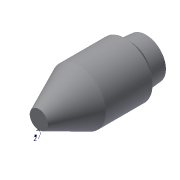
# Autodesk Inventor part: 01_Connector_T
Saved by Autodesk Inventor 2019.4 (Build 234330000, 330)
## iProperties
Created: 2021-06-01
Part Number: 01_Connector_T
Material: Generic
Document SubType Name: Modeling
Designer: diederichbenedict
Density: 1 g/cm^3
Appearance: Smooth - Red
Author: diederichbenedict
Autodesk Inventor part; units mm, degrees
ref_plane "YZ Plane" through (0, 0, 0) normal (1, 0, 0) x (0, 1, 0)
ref_plane "XZ Plane" through (0, 0, 0) normal (0, 1, 0) x (-1, 0, 0)
sketch "Sketch1" plane through (0, 0, 0) normal (1, 0, 0) x (0, 1, 0)
  line L0 (9.9, 0) -> (6.6104, -37.6)
  line L1 (11, 0) -> (11, -20)
  line L2 (-11, 0) -> (11, 0) projected
  line L3 (8.722, -6.7025) -> (0, -6.7025)
  line L4 (0, -6.7025) -> (0, 40.232)
  line L5 (0, 40.232) -> (3.984, 40.232)
  line L6 (3.984, 40.232) -> (11, 0) construction
  arc A0 (6.0149, 28.5859) -> (5.3277, 32.5264) centre (2.2587, 29.961) ccw construction
  line L7 (3.984, 40.232) -> (11.8979, 22.8363)
  line L8 (11.8979, 22.8363) -> (11.8979, 2.3768)
  line L9 (11.8979, 2.3768) -> (9.3084, 0)
  line L10 (9.3084, 0) -> (8.722, -6.7025)
  point P0 (0, 0)
  dimension "d4" = 4
  dimension "d5" = 4
  constraints: 20 end point, 3 point on line, 2 parallel, 2 perpendicular, 2 point on circle, 1 centre point, 1 horizontal, 1 vertical, 5 other
  measures "d4" distance of A0.end A0.start
  measures "d5" radius of A0
revolve "Revolution1" add sketch "Sketch1" angle 360 about axis through (0, 0, -6.7025) along (0, 0, 1)
sketch "Sketch2" plane through (0, 0, 0) normal (1, 0, 0) x (0, 1, 0)
  line L0 (-3.984, 40.232) -> (-11.8979, 22.8363) projected
  line L1 (0, 39.9349) -> (0, 14.7253)
  arc A0 (-3.984, 40.232) -> (-3.4864, 41.3256) centre (-5.4716, 41.5688) ccw
  point P0 (0, 0)
  dimension "d7" = 2
  constraints: 2 end point, 2 point on circle, 1 centre point, 1 point on line, 1 vertical
  measures "d7" radius of A0
sketch "Sketch3" plane through (0, 0, 0) normal (1, 0, 0) x (0, 1, 0)
  circle A0 centre (0, 10) radius 7.21 projected
  circle A1 centre (0, 13.2675) radius 9.5
  point P0 (0, 0)
  dimension "d8" = 19
  constraints: 1 centre point
  measures "d8" diameter of A1
ref_plane "Work Plane1" through (-17.387, -14.1299, -4.1299) normal (1, 0, 0) x (0, 1, 0)
extrude "Extrusion1" add sketch "Sketch3" against normal up to surface (17.387 mm away) contours A0 A1 | A0 A1 picked at (-1.9464, 7.9731) picked at (-0.0449, 20.8614)
sketch "Sketch4" plane through (-17.387, 0, 13.2675) normal (-1, 0, 0) x (0, 0, 1)
  circle A0 centre (0, 0) radius 9.5 projected
  circle A1 centre (0, 0) radius 7.75
  point P0 (-13.2675, 0)
  dimension "d11" = 15.5
  constraints: 1 centre point, 1 coincident
  measures "d11" diameter of A1
extrude "Extrusion2" cut sketch "Sketch4" against normal blind 15 contours A1
sketch "Sketch5" plane through (0, 0, -6.7025) normal (0, 0, -1) x (-1, 0, 0)
  circle A0 centre (0, 0) radius 9.3084 projected
  circle A1 centre (0, 0) radius 7.2846
  point P0 (0, 0)
  constraints: 1 centre point, 1 coincident
extrude "Extrusion3" cut sketch "Sketch5" against normal through all draft -5 contours A1
body "Solid1"
